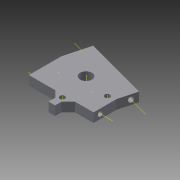
# Autodesk Inventor part: Vertex Bottom tensioner left
Saved by Autodesk Inventor 2013 (Build 170138000, 138)
## iProperties
Created: 2013-01-09
Part Number: Vertex Bottom tensioner left
Material: Generic
Document SubType Name: Modeling
Designer: Nico
Density: 1 g/cm^3
Mass: 93.0755 g
Surface Area: 267.739 cm^2
Volume: 93.0755 cm^3
Author: Nico
Autodesk Inventor part; units mm, degrees
ref_plane "YZ Plane" through (0, 0, 0) normal (1, 0, 0) x (0, 1, 0)
ref_plane "XZ Plane" through (0, 0, 0) normal (0, 1, 0) x (-1, 0, 0)
ref_plane "XY Plane" through (0, 0, 0) normal (0, 0, 1) x (1, 0, 0)
sketch "Sketch1" plane through (0, 0, 0) normal (0, 0, 1) x (1, 0, 0)
  line L0 (11.0906, 0.1113) -> (11.0906, 10.1113)
  line L1 (11.0906, 10.1113) -> (1.0906, 20.1113)
  line L2 (31.0918, 20.1126) -> (21.0906, 10.1113)
  line L3 (21.0906, 10.1113) -> (21.0906, 0.1113)
  line L4 (21.0906, 0.1113) -> (11.0906, 0.1113)
  circle A0 centre (16.0906, 16.0413) radius 3.9
  line L5 (37.1863, 89.9817) -> (4.7287, 98.6787)
  line L6 (41.216, 88.9019) -> (37.1863, 89.9817)
  circle A1 centre (31.0906, 45.1113) radius 4
  circle A2 centre (-18.9094, 45.1113) radius 4
  line L7 (1.0906, 20.1113) -> (-38.9094, 20.1113)
  line L8 (4.7287, 98.6787) -> (-28.7852, 107.6587)
  circle A3 centre (6.0906, 62.1113) radius 9
  line L9 (-38.9094, 69.8746) -> (-28.7852, 107.6587)
  line L10 (31.0918, 20.1126) -> (59.4992, 20.1126)
  line L11 (59.4992, 20.1126) -> (59.4992, 54.8735)
  line L12 (59.4992, 84.003) -> (41.216, 88.9019)
  line L13 (59.4992, 54.8735) -> (66.7815, 82.0517)
  line L14 (66.7815, 82.0517) -> (59.4992, 84.003)
  circle A4 centre (48.4066, 52.1126) radius 3.9
  line L15 (-38.9094, 69.8746) -> (-38.9094, 20.1113)
  point P0 (0, 0)
  dimension "d2" = 10
  dimension "d5" = 135
  dimension "d6" = 135
  dimension "d7" = 10
  dimension "d8" = 10
  dimension "d11" = 7.8
  dimension "d14" = 8
  dimension "d15" = 8
  dimension "d16" = 50
  dimension "d20" = 18
  dimension "d21" = 17
  dimension "d24" = 25
  dimension "d30" = 90
  dimension "d31" = 39.117
  dimension "d51" = 7.8
  dimension "d52" = 10
  dimension "d53" = 32
  dimension "d71" = 34.7609
  dimension "d72" = 25
  dimension "d73" = 25
  dimension "d74" = 5
  dimension "d75" = 49.7632
  dimension "d77" = 28.4086
  constraints: 32 end point, 5 centre point, 5 perpendicular, 3 horizontal, 2 parallel, 2 vertical, 1 collinear
  measures "d2" distance between parallel lines of L3 L0
  measures "d5" angle of L0 L1
  measures "d6" angle of L3 L2
  measures "d7" distance of L0.start L0.end
  measures "d8" distance of L2.end L3.end
  measures "d11" diameter of A0
  measures "d14" diameter of A1
  measures "d15" diameter of A2
  measures "d16" distance of A1.centre A2.centre
  measures "d20" diameter of A3
  measures "d21" vertical distance of A3.centre A2.centre
  measures "d24" horizontal distance of A2.centre A3.centre
  measures "d30" angle of L9 L8
  measures "d31" distance of L9.start L8.end
  measures "d51" diameter of A4
  measures "d52" distance from line of A4.centre L13
  measures "d53" distance from line of L10 A4.centre
  measures "d71" distance of L10.end L11.end
  measures "d72" distance from line of L7 A2.centre
  measures "d73" distance from line of L7 A1.centre
  measures "d74" distance from line of L0 A0.centre
  measures "d75" distance of L7.end L9.start
  measures "d77" distance from line of A1.centre L11
extrude "Extrusion6" add sketch "Sketch1" along normal blind 14
sketch "Sketch6" plane through (59.4992, 20.1126, 0) normal (1, 0, 0) x (0, 0, -1)
  circle A0 centre (-7, 10.2998) radius 3.8217
  line L0 (0, -20.0012) -> (-14, -20.0012) projected
  point P0 (0, -20.1126)
  dimension "d76" = 30.301
  constraints: 1 centre point
  measures "d76" distance from line of L0 A0.centre
extrude "Extrusion7" cut sketch "Sketch6" against normal blind 120
sketch "Sketch7" plane through (66.7815, 82.0517, 14) normal (0.9659, -0.2588, 0) x (0, 0, -1)
  line L0 (14, 0) -> (0, 0) projected
  circle A0 centre (7, -10) radius 3.9
  point P0 (14, -96.5401)
  dimension "d58" = 7.8
  dimension "d60" = 10
  constraints: 1 centre point
  measures "d58" diameter of A0
  measures "d60" distance from line of A0.centre L0
extrude "Extrusion8" cut sketch "Sketch7" against normal blind 120
sketch "Sketch8" plane through (0, 0, 0) normal (0, 0, -1) x (-1, 0, 0)
  circle A0 centre (-6.0906, 62.1113) radius 9 projected
  circle A1 centre (-6.0906, 62.1113) radius 11
  point P0 (0, 0)
  dimension "d63" = 22
  constraints: 1 centre point, 1 coincident
  measures "d63" diameter of A1
extrude "Extrusion9" cut sketch "Sketch8" against normal blind 7
sketch "Sketch9" plane through (0, 0, 14) normal (0, 0, 1) x (1, 0, 0)
  circle A0 centre (-18.9094, 45.1113) radius 4 projected
  circle A1 centre (31.0906, 45.1113) radius 4 projected
  point P0 (0, 0)
extrude "Extrusion10" add sketch "Sketch9" against normal blind 5
body "Solid2"
